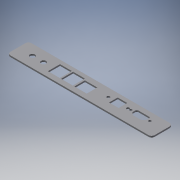
# Autodesk Inventor part: case-back
Saved by Autodesk Inventor 2017 (Build 210142000, 142)
## iProperties
Created: 2020-10-01
Part Number: case-back
Material: Generic
Document SubType Name: Modeling
Designer: jferner
Density: 1 g/cm^3
Appearance: Default
Author: jferner
Autodesk Inventor part; units mm, degrees
ref_plane "YZ Plane" through (0, 0, 0) normal (1, 0, 0) x (0, 1, 0)
ref_plane "XZ Plane" through (0, 0, 0) normal (0, 1, 0) x (-1, 0, 0)
ref_plane "XY Plane" through (0, 0, 0) normal (0, 0, 1) x (1, 0, 0)
sketch "Sketch1" plane through (0, 0, 0) normal (0, 0, 1) x (1, 0, 0)
  line L0 (-4, 0) -> (-194, 0)
  line L1 (-198, 4) -> (-198, 25)
  line L2 (-194, 29) -> (-4, 29)
  line L3 (0, 25) -> (0, 4)
  arc A0 (0, 25) -> (-4, 29) centre (-4, 25) ccw
  arc A1 (-194, 29) -> (-198, 25) centre (-194, 25) ccw
  arc A2 (-198, 4) -> (-194, 0) centre (-194, 4) ccw
  arc A3 (-4, 0) -> (0, 4) centre (-4, 4) ccw
  point P0 (0, 0)
  point P1 (-198, 0)
  point P2 (0, 29)
  dimension "d0" = 198
  dimension "d1" = 29
  dimension "d2" = 4
  constraints: 8 end point, 8 point on circle, 8 tangent, 6 point on line, 4 centre point, 3 equal radius, 2 parallel, 1 horizontal, 1 perpendicular
  measures "d0" distance of point (0, 0) point (-198, 0)
  measures "d1" distance of point (0, 29) point (0, 0)
  measures "d2" radius of A0
extrude "Extrusion1" add sketch "Sketch1" along normal blind 2
sketch "Sketch2" plane through (0, 0, 0) normal (0, 0, -1) x (-1, 0, 0)
  line L0 (95.9784, 21.4874) -> (112.8534, 21.4874)
  line L1 (112.8534, 21.4874) -> (112.8534, 7)
  line L2 (112.8534, 7) -> (95.9784, 7)
  line L3 (95.9784, 7) -> (95.9784, 21.4874)
  line L4 (194, 0) -> (4, 0) projected
  line L5 (0, 4) -> (0, 25) projected
  line L6 (115.1046, 23.6) -> (131.2046, 23.6)
  line L7 (131.2046, 23.6) -> (131.2046, 7)
  line L8 (131.2046, 7) -> (115.1046, 7)
  line L9 (115.1046, 7) -> (115.1046, 23.6)
  line L10 (133.1046, 23.6) -> (149.2046, 23.6)
  line L11 (149.2046, 23.6) -> (149.2046, 7)
  line L12 (149.2046, 7) -> (133.1046, 7)
  line L13 (133.1046, 7) -> (133.1046, 23.6)
  circle A0 centre (162.7, 14.5) radius 3.5
  circle A1 centre (178, 14.5) radius 3.5
  line L14 (198, 25) -> (198, 4) projected
  line L15 (70.05, 11.74) -> (56.95, 11.74)
  line L16 (56.95, 11.74) -> (56.95, 23.6)
  line L17 (56.95, 23.6) -> (70.05, 23.6)
  line L18 (70.05, 23.6) -> (70.05, 11.74)
  circle A2 centre (77, 17.67) radius 2
  circle A3 centre (50, 17.67) radius 2
  line L19 (63.5, 11.74) -> (63.5, 8.0383)
  line L20 (32.5145, 22.3095) -> (17.7855, 22.3095)
  line L21 (15.7855, 20.3095) -> (15.7855, 16.8274)
  line L22 (17.1974, 14.9158) -> (17.2455, 14.901)
  line L23 (18.1588, 14.3108) -> (18.6882, 13.7092)
  line L24 (20.1896, 13.0305) -> (30.1104, 13.0305)
  line L25 (31.6118, 13.7092) -> (32.1412, 14.3108)
  line L26 (33.0545, 14.901) -> (33.1026, 14.9158)
  line L27 (34.5145, 16.8274) -> (34.5145, 20.3095)
  circle A4 centre (38.3, 17.67) radius 1.75
  circle A5 centre (12, 17.67) radius 1.75
  arc A6 (33.1026, 14.9158) -> (34.5145, 16.8274) centre (32.5145, 16.8274) ccw
  arc A7 (33.0545, 14.901) -> (32.1412, 14.3108) centre (33.6426, 12.9895) ccw
  arc A8 (30.1104, 13.0305) -> (31.6118, 13.7092) centre (30.1104, 15.0305) ccw
  arc A9 (18.6882, 13.7092) -> (20.1896, 13.0305) centre (20.1896, 15.0305) ccw
  arc A10 (18.1588, 14.3108) -> (17.2455, 14.901) centre (16.6574, 12.9895) ccw
  arc A11 (15.7855, 16.8274) -> (17.1974, 14.9158) centre (17.7855, 16.8274) ccw
  arc A12 (17.7855, 22.3095) -> (15.7855, 20.3095) centre (17.7855, 20.3095) ccw
  arc A13 (34.5145, 20.3095) -> (32.5145, 22.3095) centre (32.5145, 20.3095) ccw
  point P0 (0, 0)
  point P1 (34.5145, 22.3095)
  point P2 (15.7855, 22.3095)
  point P3 (15.7855, 15.3502)
  point P4 (17.7855, 14.7349)
  point P5 (19.2855, 13.0305)
  point P6 (31.0145, 13.0305)
  point P7 (32.5145, 14.7349)
  point P8 (34.5145, 15.3502)
  dimension "d7" = 16.875
  dimension "d8" = 14.4874
  dimension "d9" = 7
  dimension "d11" = 2.2512
  dimension "d12" = 1.9
  dimension "d13" = 16.1
  dimension "d14" = 16.1
  dimension "d15" = 16.6
  dimension "d16" = 7
  dimension "d17" = 7
  dimension "d18" = 7.5
  dimension "d19" = 13.4954
  dimension "d20" = 15.3
  dimension "d21" = 20
  dimension "d22" = 13.1
  dimension "d23" = 11.86
  dimension "d24" = 0
  dimension "d26" = 27
  dimension "d27" = 4
  dimension "d28" = 13.5
  dimension "d29" = 5.93
  dimension "d30" = 9.279
  dimension "d31" = 18.729
  dimension "d32" = 107.1
  dimension "d33" = 107.1
  dimension "d34" = 138.65
  dimension "d35" = 138.65
  dimension "d36" = 2
  dimension "d37" = 2
  dimension "d38" = 3.5
  dimension "d39" = 3.5
  dimension "d40" = 3.5
  dimension "d41" = 26.3
  dimension "d42" = 3.7855
  dimension "d43" = 4.6395
  dimension "d45" = 2
  dimension "d47" = 50
  dimension "d48" = 12
  constraints: 50 end point, 17 point on line, 16 point on circle, 16 tangent, 14 centre point, 9 equal radius, 9 parallel, 5 horizontal, 5 perpendicular, 4 horizontal alignment, 2 collinear, 2 vertical, 1 midpoint
  measures "d7" distance of L1.end L2.end
  measures "d8" distance of L2.end L0.start
  measures "d9" distance between parallel lines of L4 L2
  measures "d11" distance between parallel lines of L9 L1
  measures "d12" distance between parallel lines of L13 L7
  measures "d13" distance between parallel lines of L7 L9
  measures "d14" distance between parallel lines of L11 L13
  measures "d15" distance between parallel lines of L10 L12
  measures "d16" diameter of A0
  measures "d17" diameter of A1
  measures "d18" distance from line of L12 A0.centre
  measures "d19" distance from line of A0.centre L11
  measures "d20" distance of A1.centre A0.centre
  measures "d21" distance from line of L14 A1.centre
  measures "d22" distance of L16.end L17.end
  measures "d23" distance of L15.end L16.end
  measures "d24" distance between parallel lines of L6 L17
  measures "d26" distance of A3.centre A2.centre
  measures "d27" diameter of A2
  measures "d28" distance from line of L19 A2.centre
  measures "d29" distance from line of L15 A2.centre
  measures "d30" distance between parallel lines of L20 L24
  measures "d31" distance between parallel lines of L21 L27
  measures "d32" angle of L21 L22
  measures "d33" angle of L27 L26
  measures "d34" angle of L27 L25
  measures "d35" angle of L21 L23
  measures "d36" distance from line of point (32.515, 14.735) L27
  measures "d37" distance from line of L21 point (17.786, 14.735)
  measures "d38" distance from line of point (31.015, 13.031) L27
  measures "d39" distance from line of point (19.286, 13.031) L21
  measures "d40" diameter of A4
  measures "d41" distance of A5.centre A4.centre
  measures "d42" distance from line of L21 A5.centre
  measures "d43" distance from line of L20 A5.centre
  measures "d45" radius of A6
  measures "d47" distance from line of L5 A3.centre
  measures "d48" distance from line of L5 A5.centre
extrude "Extrusion2" cut sketch "Sketch2" against normal through all
equation "\"d0\" = caseBottomWidth - thickness"
equation "\"d1\" = -thickness + 2 * caseBottomHeight - lipHeight"
equation "\"d2\" = filletMid"
equation "\"d3\" = thickness"
equation "\"d14\" = d13"
equation "\"d21\" = offsetFromSideOfCase"
equation "\"d28\" = 0.5 * d26"
equation "\"d29\" = 0.5 * d23"
equation "\"d33\" = d32"
equation "\"d35\" = d34"
equation "\"d37\" = d36"
equation "\"d39\" = d38"
equation "\"d42\" = -0.5 * d31 + 0.5 * d41"
equation "\"d43\" = 0.5 * d30"
equation "\"d5\" = thickness"
equation "\"filletMid\" = 4"
equation "\"thickness\" = 2"
equation "\"offsetFromSideOfCase\" = 20"
equation "\"caseBottomWidth\" = 200"
equation "\"caseBottomHeight\" = 16"
equation "\"lipHeight\" = 1"
body "Solid1"
